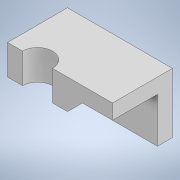
# Autodesk Inventor part: 件28
Saved by Autodesk Inventor 2020 (Build 240168000, 168)
## iProperties
Created: 2020-10-30
Part Number: 件28
Material: 一般
Document SubType Name: Modeling
Designer: USER
Density: 1 g/cm^3
Appearance: 預設
Author: USER
Autodesk Inventor part; units mm, degrees
ref_plane "YZ Plane" through (0, 0, 0) normal (1, 0, 0) x (0, 1, 0)
ref_plane "XZ Plane" through (0, 0, 0) normal (0, 1, 0) x (-1, 0, 0)
ref_plane "XY Plane" through (0, 0, 0) normal (0, 0, 1) x (1, 0, 0)
sketch "草圖1" plane through (0, 0, 0) normal (0, 0, 1) x (1, 0, 0)
  line L0 (35, -20) -> (-35, -20)
  line L1 (-35, -20) -> (-35, 20)
  line L2 (-35, 20) -> (35, 20)
  line L3 (35, 20) -> (35, -20)
  line L4 (35, -20) -> (-35, 20) construction
  line L5 (-35, -20) -> (35, 20) construction
  point P0 (0, 0)
  dimension "d0" = 70
  dimension "d1" = 40
  constraints: 12 end point, 2 midpoint, 2 parallel, 1 horizontal, 1 perpendicular
  measures "d0" distance between parallel lines of L3 L1
  measures "d1" distance between parallel lines of L0 L2
extrude "擠出1" add sketch "草圖1" along normal blind 10
sketch "草圖2" plane through (0, 0, 10) normal (0, 0, 1) x (1, 0, 0)
  line L0 (35, 20) -> (-35, 20) projected
  line L1 (-35, 20) -> (5, 20)
  line L2 (5, 20) -> (5, 0)
  line L3 (5, 0) -> (-35, 0)
  line L4 (-35, 0) -> (-35, 20)
  line L5 (35, 20) -> (15, 20)
  line L6 (15, 20) -> (15, 10)
  line L7 (15, 10) -> (35, 10)
  line L8 (35, 10) -> (35, 20)
  point P0 (0, 0)
  point P1 (5, 20)
  dimension "d4" = 20
  dimension "d5" = 10
  dimension "d6" = 40
  dimension "d7" = 20
  constraints: 16 end point, 4 parallel, 2 horizontal, 2 perpendicular
  measures "d4" distance between parallel lines of L8 L6
  measures "d5" distance between parallel lines of L7 L0
  measures "d6" distance between parallel lines of L2 L4
  measures "d7" distance between parallel lines of L0 L3
extrude "擠出2" add sketch "草圖2" along normal blind 30
sketch "草圖3" plane through (-35, 0, 10) normal (0, -1, 0) x (1, 0, 0)
  circle A0 centre (20, 30) radius 10
  line L0 (0, 0) -> (0, 30) projected
  line L1 (0, 0) -> (70, 0) projected
  point P0 (35, -10)
  dimension "d14" = 20
  dimension "d15" = 20
  dimension "d16" = 30
  constraints: 1 centre point
  measures "d14" distance from line of A0.centre L0
  measures "d15" diameter of A0
  measures "d16" distance from line of L1 A0.centre
extrude "擠出3" cut sketch "草圖3" against normal blind 30
sketch "草圖4" plane through (5, 0, 10) normal (1, 0, 0) x (0, 0, -1)
  line L0 (-30, 20) -> (-30, 0) projected
  line L1 (-30, 0) -> (-0.078, 0)
  line L2 (-0.078, 0) -> (-0.078, 20)
  line L3 (-0.078, 20) -> (-30, 20)
  line L4 (-30, 20) -> (-30, 0)
  point P0 (10, 0)
  constraints: 8 end point, 2 parallel, 1 horizontal, 1 perpendicular
loft "斷面混成2" add section 1 edges at (15, 15, 10) (15, 10, 25) (15, 15, 40) (15, 20, 25) section 2 edges at (5, 10, 10) (5, 20, 25) (5, 10, 40) (5, 0, 25)
